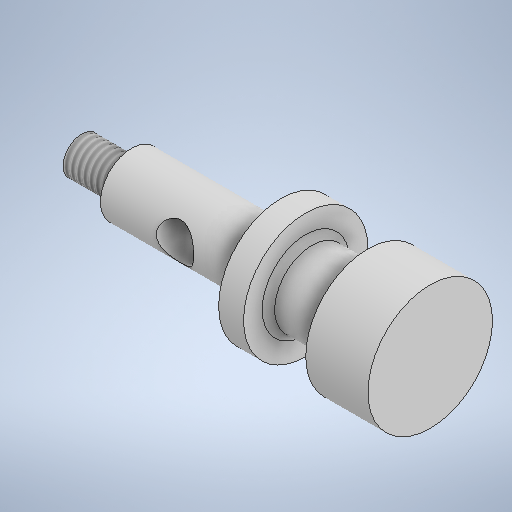
# Autodesk Inventor part: 141
Saved by Autodesk Inventor 2025.1 (Build 291241000, 241)
## iProperties
Created: 2024-08-05
Part Number: 141
Material: Generisch
Document SubType Name: Modeling
Designer: ffogue
Density: 1 g/cm^3
Appearance: Vorgabe
Author: ffogue
Autodesk Inventor part; units mm, degrees
ref_plane "YZ Plane" through (0, 0, 0) normal (1, 0, 0) x (0, 1, 0)
ref_plane "XY Plane" through (0, 0, 0) normal (0, 0, 1) x (1, 0, 0)
sketch "Sketch1" plane through (0, 0, 0) normal (0, 0, 1) x (1, 0, 0)
  line L0 (0, 0) -> (0, 1.5)
  line L1 (0, 1.5) -> (4, 1.5)
  line L2 (4, 1.5) -> (4, 2.5)
  line L3 (4, 2.5) -> (16, 2.5)
  line L4 (16, 2.5) -> (16, 5)
  line L5 (16, 5) -> (18, 5)
  line L6 (18, 5) -> (18, 3)
  line L7 (18, 3) -> (23, 3)
  line L8 (23, 3) -> (23, 5)
  line L9 (23, 5) -> (28, 5)
  line L10 (28, 5) -> (28, 0)
  line L11 (28, 0) -> (0, 0)
  dimension "d0" = 28
  dimension "d1" = 5
  dimension "d2" = 5
  dimension "d3" = 2
  dimension "d4" = 12
  dimension "d5" = 3
  dimension "d6" = 5
  dimension "d7" = 10
  dimension "d8" = 6
  constraints: 24 end point, 9 perpendicular, 2 point on line, 1 parallel, 1 vertical
  measures "d0" distance of L10.end L0.start
  measures "d1" distance of L8.end L9.end
  measures "d2" distance of L6.end L7.end
  measures "d3" distance of L4.end L5.end
  measures "d4" distance of L2.end L3.end
  measures "d5" diameter of L1 L11
  measures "d6" diameter of L3 L11
  measures "d7" diameter of L9 L11
  measures "d8" diameter of L7 L11
revolve "Revolution1" add sketch "Sketch1" angle 360 about axis through (28, 0, 0) along (-1, 0, 0)
ref_plane "Work Plane1" through (0, 2.5, 0) normal (0, 1, 0) x (-1, 0, 0)
sketch "Sketch2" plane through (0, 2.5, 0) normal (0, 1, 0) x (-1, 0, 0)
  line L0 (-4, -2.5) -> (-4, 2.5) projected
  point P0 (0, 0)
  point P1 (-10, 0)
  dimension "d11" = 6
  constraints: 1 horizontal alignment
  measures "d11" distance from line of point (-10, 0) L0
hole "Hole1" at (10, 2.5, 0) direction (0, -1, 0) diameter 3 end through all
thread "Thread1" size "M3x0.5" class "6g" standard "ISO Metric profile" length 10
fillet "Fillet1" radius 0.5 2 edges at (18, -3, 0) (23, -3, 0)
sketch "Sketch4" plane through (0, 2.5, 0) normal (0, 1, 0) x (-1, 0, 0)
  line L0 (-28, -5) -> (-28, 5) projected
  point P0 (0, 0)
  point P1 (-25.5, 0)
  point P2 (-28, 0)
  dimension "d22" = 2.5
  constraints: 1 horizontal alignment, 1 midpoint
  measures "d22" distance of point (-28, 0) point (-25.5, 0)
hole "Hole2" at (25.5, 2.5, 0) direction (0, 1, 0) diameter 3 end through all
thread "Thread2" size "M3x0.5" class "6H" standard "ISO Metric profile" length 10
body "Solid1"
